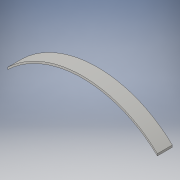
# Autodesk Inventor part: Clip
Saved by Autodesk Inventor 2016 (Build 200138000, 138)
## iProperties
Created: 2016-08-17
Part Number: Clip
Material: Generic
Document SubType Name: Modeling
Designer: yash
Density: 1 g/cm^3
Appearance: Default
Author: yash
Autodesk Inventor part; units mm, degrees
ref_plane "YZ Plane" through (0, 0, 0) normal (1, 0, 0) x (0, 1, 0)
ref_plane "XZ Plane" through (0, 0, 0) normal (0, 1, 0) x (-1, 0, 0)
ref_plane "XY Plane" through (0, 0, 0) normal (0, 0, 1) x (1, 0, 0)
sketch "Sketch1" plane through (0, 0, 0) normal (0, 0, 1) x (1, 0, 0)
  line L0 (0, 0) -> (127, 0) construction
  line L1 (0, 0) -> (127, 0) construction
  line L2 (0, 0) -> (63.5, 0) construction
  line L3 (0, 0) -> (63.5, 0) construction
  line L4 (63.5, 0) -> (63.5, 25.4) construction
  arc A0 (127, 0) -> (0, 0) centre (63.5, -66.675) ccw
  line L5 (63.5, 25.4) -> (63.5, 27.1272) construction
  line L6 (0, 0) -> (0, 1.7272) construction
  line L7 (127, 0) -> (127, 1.7272) construction
  arc A1 (127, 1.7272) -> (0, 1.7272) centre (63.5, -64.9478) ccw
  line L8 (0, 0) -> (0, 1.7272)
  line L9 (127, 0) -> (127, 1.7272)
  dimension "d4" = 127
  dimension "d5" = 63.5
  dimension "d6" = 0
  dimension "d7" = 25.4
  dimension "d8" = 1.7272
  dimension "d9" = 1.7272
  dimension "d10" = 1.7272
  constraints: 20 end point, 6 point on circle, 5 vertical, 4 horizontal, 2 centre point, 2 collinear, 1 parallel
  measures "d4" distance of L0.start L0.end
  measures "d5" distance of L0.start L2.end
  measures "d6" distance between parallel lines of L2 L3
  measures "d7" distance of L3.end L4.end
  measures "d8" distance of L4.end L5.end
  measures "d9" distance of L0.start L6.end
  measures "d10" distance of L1.end L7.end
extrude "Extrusion1" add sketch "Sketch1" along normal blind 12.7
body "Solid1"
